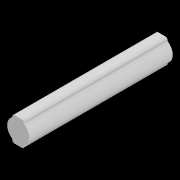
# Autodesk Inventor part: Axel_parametriserad_02
Saved by Autodesk Inventor 2020 (Build 240168000, 168)
## iProperties
Created: 2020-11-21
Part Number: Axel_parametriserad_02
Material: Generic
Document SubType Name: Modeling
Designer: Gottfrid
Density: 1 g/cm^3
Appearance: Default
Author: Gottfrid
Autodesk Inventor part; units mm, degrees
ref_plane "YZ Plane" through (0, 0, 0) normal (1, 0, 0) x (0, 1, 0)
ref_plane "XZ Plane" through (0, 0, 0) normal (0, 1, 0) x (-1, 0, 0)
ref_plane "XY Plane" through (0, 0, 0) normal (0, 0, 1) x (1, 0, 0)
sketch "Sketch1" plane through (0, 0, 0) normal (0, 0, 1) x (1, 0, 0)
  circle A0 centre (0, 0) radius 3.2
  line L0 (1.1569, -3.5962) -> (-1.1569, -3.5962)
  line L1 (-1.6569, -3.0962) -> (-1.6569, 3.0962)
  line L2 (-1.1569, 3.5962) -> (1.1569, 3.5962)
  line L3 (1.6569, 3.0962) -> (1.6569, -3.0962)
  line L4 (1.6569, -3.5962) -> (-1.6569, 3.5962) construction
  line L5 (-1.6569, -3.5962) -> (1.6569, 3.5962) construction
  arc A1 (-1.1569, 3.5962) -> (-1.6569, 3.0962) centre (-1.1569, 3.0962) ccw
  arc A2 (1.6569, 3.0962) -> (1.1569, 3.5962) centre (1.1569, 3.0962) ccw
  arc A3 (1.1569, -3.5962) -> (1.6569, -3.0962) centre (1.1569, -3.0962) ccw
  arc A4 (-1.6569, -3.0962) -> (-1.1569, -3.5962) centre (-1.1569, -3.0962) ccw
  point P0 (-1.6569, 3.5962)
  point P1 (1.6569, 3.5962)
  point P2 (1.6569, -3.5962)
  point P3 (1.6569, -3.5962)
  point P4 (1.6569, 2.7377)
  point P5 (-1.6569, 2.7377)
  point P6 (-1.6569, -2.7377)
  point P7 (1.6569, -2.7377)
  point P8 (-1.6569, 3.5962)
  point P9 (-1.6569, 3.5962)
  point P10 (1.6569, 3.5962)
  point P11 (1.6569, -3.5962)
  point P12 (1.6569, -3.5962)
  point P13 (-1.6569, -3.5962)
  dimension "d0" = 6.4
  dimension "d1" = 7.1923
  dimension "d2" = 3.3137
  dimension "d7" = 0.5
  constraints: 24 point on line, 12 end point, 9 horizontal, 8 point on circle, 8 tangent, 8 vertical, 5 centre point, 3 equal radius, 2 midpoint, 2 parallel, 1 coincident, 1 perpendicular, 32 other
  measures "d0" diameter of A0
  measures "d1" distance between parallel lines of L0 L2
  measures "d2" distance between parallel lines of L3 L1
  measures "d7" radius of A1
extrude "Extrusion1" add sketch "Sketch1" along normal blind 42
equation "\"d0\" = D_inreRing_i - d_toleransAxel"
equation "\"d7\" = r_filletAxel"
equation "\"d4\" = h_axel"
equation "\"d_toleransAxel\" = 0.1"
equation "\"h_axel\" = 42"
equation "\"D_inreRing_i\" = 6.5"
equation "\"r_filletAxel\" = 0.5"
body "Solid1"
